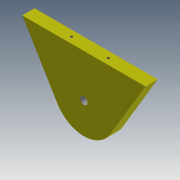
# Autodesk Inventor part: stojan2
Saved by Autodesk Inventor 2013 (Build 170138000, 138)
## iProperties
Created: 2013-06-04
Part Number: stojan2
Material: Generic
Document SubType Name: Modeling
Designer: idle-rug
Density: 1 g/cm^3
Author: idle-rug
Autodesk Inventor part; units mm, degrees
ref_plane "YZ Plane" through (0, 0, 0) normal (1, 0, 0) x (0, 1, 0)
ref_plane "XZ Plane" through (0, 0, 0) normal (0, 1, 0) x (-1, 0, 0)
ref_plane "XY Plane" through (0, 0, 0) normal (0, 0, 1) x (1, 0, 0)
sketch "Sketch1" plane through (0, 0, 0) normal (0, 1, 0) x (-1, 0, 0)
  circle A0 centre (0, -35) radius 25
  line L0 (0, 0) -> (50, 0)
  line L1 (50, 0) -> (-50, 0)
  line L2 (21.4679, -47.8113) -> (50, 0)
  line L3 (-21.4679, -47.8113) -> (-50, 0)
  circle A1 centre (0, -35) radius 3
  dimension "d4" = 50
  dimension "d5" = 50
  dimension "d6" = 100
  dimension "d7" = 6
  constraints: 8 end point, 2 centre point, 2 coincident, 2 point on circle, 2 tangent, 1 collinear, 1 horizontal, 1 point on line, 1 other
  measures "d4" diameter of A0
  measures "d5" distance of L0.start L0.end
  measures "d6" distance of L0.end L1.end
  measures "d7" diameter of A1
extrude "Extrusion1" add sketch "Sketch1" along normal blind 10
sketch "Sketch2" plane through (-50, 0, 0) normal (0, 0, 1) x (1, 0, 0)
  line L0 (0, 10) -> (100, 10) projected
  line L1 (0, 10) -> (50, 10)
  line L2 (50, 10) -> (50, 0)
  circle A0 centre (35, 5) radius 1
  circle A1 centre (65, 5) radius 1
  dimension "d11" = 2
  dimension "d12" = 2
  constraints: 4 end point, 2 centre point, 1 midpoint, 1 perpendicular
  measures "d11" diameter of A0
  measures "d12" diameter of A1
extrude "Extrusion2" cut sketch "Sketch2" against normal blind 10
body "Solid1"
